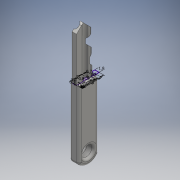
# Autodesk Inventor part: kms01
Saved by Autodesk Inventor 2016 (Build 200138000, 138)
## iProperties
Created: 2016-08-11
Part Number: kms01
Material: Generic
Document SubType Name: Modeling
Designer: Chris
Density: 1 g/cm^3
Appearance: Default
Author: Chris
Autodesk Inventor part; units mm, degrees
ref_plane "YZ Plane" through (0, 0, 0) normal (1, 0, 0) x (0, 1, 0)
ref_plane "XZ Plane" through (0, 0, 0) normal (0, 1, 0) x (-1, 0, 0)
ref_plane "XY Plane" through (0, 0, 0) normal (0, 0, 1) x (1, 0, 0)
sketch "Sketch1" plane through (0, 0, 0) normal (0, 0, 1) x (1, 0, 0)
  line L0 (-0.9, 0) -> (0.9, 0)
  line L1 (0.9, 0) -> (0.9, 9.3)
  line L2 (0.9, 9.3) -> (-0.9, 9.3)
  line L3 (-0.9, 9.3) -> (-0.9, 0)
  arc A0 (-0.9, 0.7) -> (-0.9, 2.8) centre (-0.8511, 1.75) ccw
  arc A1 (0.9, 5) -> (0.9, 3) centre (0.9, 4) ccw
  arc A2 (-0.9, 5) -> (-0.3932, 7) centre (-0.876, 6.0581) ccw
  line L4 (0.9, 7) -> (0.4, 7)
  line L5 (0.4, 7) -> (0.9, 6)
  line L6 (0.4, 7) -> (0.4, 8)
  line L7 (0.4, 8) -> (0.9, 8)
  line L8 (-0.9, 8) -> (-0.3, 8)
  line L9 (-0.3, 8) -> (-0.3, 6.9461)
  point P0 (0, 0)
  point P1 (0, 0)
  point P2 (0.2, 1.75)
  point P3 (-0.1, 4)
  point P4 (0.15, 5.7981)
  dimension "d0" = 1.8
  dimension "d1" = 9.3
  dimension "d18" = 2.8
  dimension "d19" = 0.7
  dimension "d20" = 0.7
  dimension "d21" = 3
  dimension "d22" = 5
  dimension "d23" = 0.8
  dimension "d24" = 5
  dimension "d25" = 7
  dimension "d26" = 0.75
  dimension "d27" = 7
  dimension "d28" = 6
  dimension "d29" = 0.5
  dimension "d34" = 0.7
  dimension "d35" = 8
  constraints: 20 end point, 11 point on line, 10 point on circle, 3 centre point, 3 perpendicular, 2 horizontal, 2 parallel, 1 coincident, 1 midpoint, 1 vertical
  measures "d0" distance of L2.end L1.end
  measures "d1" distance of L0.end L1.end
  measures "d18" distance from line of L0 A0.end
  measures "d19" distance of L0.start A0.start
  measures "d20" distance from line of L1 point (0.2, 1.75)
  measures "d21" distance from line of L0 A1.end
  measures "d22" distance from line of L0 A1.start
  measures "d23" distance from line of L3 point (-0.1, 4)
  measures "d24" vertical distance of point (0, 0) A2.start
  measures "d25" vertical distance of point (0, 0) A2.end
  measures "d26" distance from line of L1 point (0.15, 5.798)
  measures "d27" vertical distance of point (0, 0) L4.start
  measures "d28" vertical distance of point (0, 0) L5.end
  measures "d29" distance of L4.start L4.end
  measures "d34" distance between parallel lines of L6 L9
  measures "d35" distance from line of point (0, 0) L7
sketch "Sketch2" plane through (0, 0, 0) normal (1, 0, 0) x (0, 1, 0)
  line L0 (6.8, 0) -> (6.8, 3.6)
  line L1 (6.8, 3.6) -> (5.5, 4.9)
  line L2 (6, 17.75) -> (2.75, 21)
  line L3 (2.75, 21) -> (0, 18.25)
  line L4 (0, 18.25) -> (0, 0)
  line L5 (0, 0) -> (6.8, 0)
  line L6 (6, 16.5) -> (0, 16.5) construction
  line L7 (4.55, 13) -> (0, 13) construction
  line L8 (6.35, 9.5) -> (0, 9.5) construction
  line L9 (5.5, 6) -> (0, 6) construction
  arc A0 (3.4571, 20.2929) -> (2.0429, 20.2929) centre (2.75, 19.5858) ccw
  line L10 (5.5, 7.325) -> (5.5, 4.9)
  line L11 (6.35, 10.35) -> (6.35, 8.175)
  line L12 (4.55, 14.025) -> (4.55, 12.15)
  line L13 (6, 17.75) -> (6, 15.475)
  line L14 (6, 15.475) -> (4.55, 14.025)
  line L15 (4.55, 12.15) -> (6.35, 10.35)
  line L16 (6.35, 8.175) -> (5.5, 7.325)
  line L17 (1.375, 6) -> (1.375, 9.5) construction
  line L18 (1.375, 9.5) -> (1.375, 13) construction
  line L19 (1.375, 13) -> (1.375, 9.5) construction
  line L20 (1.375, 13) -> (1.375, 16.5) construction
  line L21 (1.375, 6) -> (1.375, 2.5) construction
  point P0 (1.375, 11.25)
  point P1 (1.375, 7.75)
  point P2 (5.45, 11.25)
  point P3 (5.925, 7.75)
  point P4 (5.275, 14.75)
  point P5 (1.375, 14.75)
  point P6 (6.15, 4.25)
  point P7 (1.375, 4.25)
  dimension "d3" = 135
  dimension "d6" = 6.8
  dimension "d7" = 5.5
  dimension "d8" = 6.35
  dimension "d9" = 4.55
  dimension "d10" = 6
  dimension "d11" = 6
  dimension "d12" = 9.5
  dimension "d13" = 13
  dimension "d14" = 16.5
  dimension "d15" = 21
  dimension "d16" = 2.75
  dimension "d17" = 1
  dimension "d39" = 135
  constraints: 48 end point, 16 point on line, 9 midpoint, 6 perpendicular, 6 vertical, 4 horizontal alignment, 4 parallel, 2 point on circle, 2 tangent, 1 centre point, 1 collinear, 1 horizontal
  measures "d3" angle of L1 L0
  measures "d6" distance between parallel lines of L4 L0
  measures "d7" distance of L9.end L9.start
  measures "d8" distance of L8.end L8.start
  measures "d9" distance of L7.end L7.start
  measures "d10" distance of L6.end L6.start
  measures "d11" distance from line of L9 L4.end
  measures "d12" distance from line of L4.end L8
  measures "d13" distance from line of L4.end L7
  measures "d14" distance from line of L4.end L6
  measures "d15" vertical distance of L4.end L2.end
  measures "d16" distance from line of L2.end L4
  measures "d17" radius of A0
  measures "d39" angle of L10 L16
extrude "Extrusion1" add sketch "Sketch1" along normal up to surface (21 mm away) contours L3 A0 A2 L9 L8 L2 L1 L7 L6 L5 A1 L0
fillet "Fillet1" radius 1 7 edges at (0.9, 5, 10.5) (0.9, 6, 10.5) (-0.9, 2.8, 10.5) (0.9, 3, 10.5) (-0.9, 5, 10.5) (-0.3, 6.9461, 10.5) (0.4, 7, 10.5)
extrude "Extrusion2" cut sketch "Sketch2" along normal through all both and the other way through all contours L5 L4 L3 A0 L2 L13 L14 L12 L15 L11 L16 L10 L1 L0 keep common part
sketch "Sketch3" plane through (0, 0, 0) normal (0, 0, 1) x (1, 0, 0)
  line L0 (0.9, 0) -> (0.9, 5.7639) projected
  line L1 (-2, 8) -> (2, 8)
  line L2 (2, 8) -> (2, 0)
  line L3 (2, 0) -> (-2, 0)
  line L4 (-2, 0) -> (-2, 8)
  line L5 (-0.9, 0) -> (0.9, 0) projected
  line L6 (0.4, 8) -> (0.9, 8) projected
  point P0 (0, 0)
  point P1 (0.9, 3)
  point P2 (0, 0)
  dimension "d47" = 4
  constraints: 8 end point, 2 midpoint, 2 parallel, 1 collinear, 1 horizontal, 1 perpendicular
  measures "d47" distance of L1.start L1.end
extrude "Extrusion3" add sketch "Sketch3" against normal blind 30
sketch "Sketch4" plane through (-2, 0, 0) normal (-1, 0, 0) x (0, 0, 1)
  circle A0 centre (-25.25, 4) radius 2.25
  line L0 (-23, 8) -> (0, 8) construction
  line L1 (0, 8) -> (0, 0) construction
  line L2 (0, 0) -> (-23, 0) construction
  line L3 (-23, 0) -> (-23, 8) construction
  line L4 (-30, 0) -> (-30, 8) projected
  line L5 (0, 0) -> (-30, 0) projected
  line L6 (0, 8) -> (-30, 8) projected
  arc A1 (-27.8117, 8) -> (-27.8117, 0) centre (-25.25, 4) ccw
  spline S0 degree 2 poles (-17.6667, 1.662) (-17.6667, 1.6197) (-17.7089, 1.554) (-17.8263, 1.5117) (-18.0376, 1.4883) (-18.1925, 1.4883) knots 0 0 0 1 2 3 4 4 4
  spline S1 degree 2 poles (-18.1925, 1.4883) (-18.4413, 1.4883) (-18.662, 1.5258) (-18.7559, 1.6056) (-18.784, 1.6573) knots 0 0 0 1 2 3 3 3
  line L7 (-18.784, 1.6573) -> (-20.2911, 4.0188)
  line L8 (-20.2911, 4.0188) -> (-20.2911, 1.6573)
  spline S2 degree 2 poles (-20.2911, 1.6573) (-20.2911, 1.615) (-20.338, 1.554) (-20.4507, 1.5117) (-20.6432, 1.4883) (-20.7934, 1.4883) knots 0 0 0 1 2 3 4 4 4
  spline S3 degree 2 poles (-20.7934, 1.4883) (-20.939, 1.4883) (-21.1362, 1.5117) (-21.2488, 1.554) (-21.3005, 1.615) (-21.3005, 1.6573) knots 0 0 0 1 2 3 4 4 4
  line L9 (-21.3005, 1.6573) -> (-21.3005, 6.3474)
  spline S4 degree 2 poles (-21.3005, 6.3474) (-21.3005, 6.3897) (-21.2488, 6.4507) (-21.1362, 6.4883) (-20.939, 6.5117) (-20.7934, 6.5117) knots 0 0 0 1 2 3 4 4 4
  spline S5 degree 2 poles (-20.7934, 6.5117) (-20.6432, 6.5117) (-20.4507, 6.4883) (-20.338, 6.4507) (-20.2911, 6.3897) (-20.2911, 6.3474) knots 0 0 0 1 2 3 4 4 4
  line L10 (-20.2911, 6.3474) -> (-20.2911, 4.2254)
  line L11 (-20.2911, 4.2254) -> (-18.831, 6.3427)
  spline S6 degree 2 poles (-18.831, 6.3427) (-18.8028, 6.3944) (-18.7277, 6.4601) (-18.6056, 6.4977) (-18.4131, 6.5117) (-18.2629, 6.5117) knots 0 0 0 1 2 3 4 4 4
  spline S7 degree 2 poles (-18.2629, 6.5117) (-18.108, 6.5117) (-17.9061, 6.4883) (-17.7887, 6.446) (-17.7418, 6.385) (-17.7418, 6.3474) knots 0 0 0 1 2 3 4 4 4
  spline S8 degree 2 poles (-17.7418, 6.3474) (-17.7418, 6.2817) (-17.8122, 6.1408) (-17.9061, 5.9906) knots 0 0 0 1 2 2 2
  line L12 (-17.9061, 5.9906) -> (-19.277, 4.2019)
  line L13 (-19.277, 4.2019) -> (-17.784, 1.9531)
  spline S9 degree 2 poles (-17.784, 1.9531) (-17.6995, 1.7981) (-17.6667, 1.6901) (-17.6667, 1.662) knots 0 0 0 1 2 2 2
  spline S10 degree 2 poles (-11.1878, 1.6479) (-11.1878, 1.6103) (-11.23, 1.5493) (-11.3427, 1.5117) (-11.5258, 1.4883) (-11.6667, 1.4883) knots 0 0 0 1 2 3 4 4 4
  spline S11 degree 2 poles (-11.6667, 1.4883) (-11.8075, 1.4883) (-11.9906, 1.5117) (-12.0986, 1.5493) (-12.1455, 1.6103) (-12.1455, 1.6479) knots 0 0 0 1 2 3 4 4 4
  line L14 (-12.1455, 1.6479) -> (-12.1455, 5.6995)
  line L15 (-12.1455, 5.6995) -> (-12.1549, 5.6995)
  line L16 (-12.1549, 5.6995) -> (-13.5962, 1.6526)
  spline S12 degree 2 poles (-13.5962, 1.6526) (-13.6103, 1.6056) (-13.6808, 1.5399) (-13.7981, 1.4977) (-13.9859, 1.4883) (-14.1174, 1.4883) knots 0 0 0 1 2 3 4 4 4
  spline S13 degree 2 poles (-14.1174, 1.4883) (-14.2441, 1.4883) (-14.4319, 1.507) (-14.5493, 1.5493) (-14.6197, 1.6103) (-14.6291, 1.6526) knots 0 0 0 1 2 3 4 4 4
  line L17 (-14.6291, 1.6526) -> (-16.0235, 5.6995)
  line L18 (-16.0235, 5.6995) -> (-16.0329, 5.6995)
  line L19 (-16.0329, 5.6995) -> (-16.0329, 1.6479)
  spline S14 degree 2 poles (-16.0329, 1.6479) (-16.0329, 1.6103) (-16.0751, 1.5493) (-16.1925, 1.5117) (-16.3709, 1.4883) (-16.5117, 1.4883) knots 0 0 0 1 2 3 4 4 4
  spline S15 degree 2 poles (-16.5117, 1.4883) (-16.6526, 1.4883) (-16.8357, 1.5117) (-16.9484, 1.5493) (-16.9906, 1.6103) (-16.9906, 1.6479) knots 0 0 0 1 2 3 4 4 4
  line L20 (-16.9906, 1.6479) -> (-16.9906, 6.0845)
  spline S16 degree 2 poles (-16.9906, 6.0845) (-16.9906, 6.2817) (-16.784, 6.4883) (-16.6103, 6.4883) knots 0 0 0 1 2 2 2
  line L21 (-16.6103, 6.4883) -> (-15.9484, 6.4883)
  spline S17 degree 2 poles (-15.9484, 6.4883) (-15.77, 6.4883) (-15.5164, 6.4319) (-15.3333, 6.2958) (-15.2113, 6.0751) (-15.1643, 5.9155) knots 0 0 0 1 2 3 4 4 4
  line L22 (-15.1643, 5.9155) -> (-14.0845, 2.9484)
  line L23 (-14.0845, 2.9484) -> (-14.0704, 2.9484)
  line L24 (-14.0704, 2.9484) -> (-12.9531, 5.9061)
  spline S18 degree 2 poles (-12.9531, 5.9061) (-12.9014, 6.0704) (-12.784, 6.2911) (-12.6244, 6.4319) (-12.4131, 6.4883) (-12.2676, 6.4883) knots 0 0 0 1 2 3 4 4 4
  line L25 (-12.2676, 6.4883) -> (-11.5869, 6.4883)
  spline S19 degree 2 poles (-11.5869, 6.4883) (-11.4836, 6.4883) (-11.3333, 6.4366) (-11.2394, 6.3286) (-11.1878, 6.1784) (-11.1878, 6.0845) knots 0 0 0 1 2 3 4 4 4
  line L26 (-11.1878, 6.0845) -> (-11.1878, 1.6479)
  spline S20 degree 2 poles (-7.1549, 3.0047) (-7.1549, 2.6103) (-7.446, 2.0188) (-7.9484, 1.6244) (-8.615, 1.4225) (-8.9953, 1.4225) knots 0 0 0 1 2 3 4 4 4
  spline S21 degree 2 poles (-8.9953, 1.4225) (-9.2535, 1.4225) (-9.6948, 1.507) (-10.0329, 1.6291) (-10.2629, 1.7606) (-10.3615, 1.8592) (-10.4038, 2.0469) (-10.4038, 2.2254) knots 0 0 0 1 2 3 4 5 6 6 6
  spline S22 degree 2 poles (-10.4038, 2.2254) (-10.4038, 2.3427) (-10.3897, 2.507) (-10.3521, 2.6056) (-10.2958, 2.6479) (-10.2582, 2.6479) knots 0 0 0 1 2 3 4 4 4
  spline S23 degree 2 poles (-10.2582, 2.6479) (-10.2019, 2.6479) (-10.0094, 2.5211) (-9.6995, 2.3662) (-9.2723, 2.2394) (-8.9953, 2.2394) knots 0 0 0 1 2 3 4 4 4
  spline S24 degree 2 poles (-8.9953, 2.2394) (-8.8075, 2.2394) (-8.5164, 2.3286) (-8.3146, 2.4883) (-8.2066, 2.7277) (-8.2066, 2.8732) knots 0 0 0 1 2 3 4 4 4
  spline S25 degree 2 poles (-8.2066, 2.8732) (-8.2066, 3.0423) (-8.3897, 3.2864) (-8.6854, 3.4742) (-9.061, 3.6385) (-9.4648, 3.8216) (-9.8404, 4.0563) (-10.1362, 4.385) (-10.3192, 4.831) (-10.3192, 5.1408) knots 0 0 0 1 2 3 4 5 6 7 8 8 8
  spline S26 degree 2 poles (-10.3192, 5.1408) (-10.3192, 5.5023) (-10.0516, 6.0423) (-9.6056, 6.3991) (-8.9906, 6.5775) (-8.6479, 6.5775) knots 0 0 0 1 2 3 4 4 4
  spline S27 degree 2 poles (-8.6479, 6.5775) (-8.4742, 6.5775) (-8.1174, 6.5258) (-7.8122, 6.4319) (-7.5728, 6.3146) (-7.493, 6.2394) (-7.4695, 6.1878) (-7.4507, 6.0986) (-7.4413, 5.9624) (-7.4413, 5.8638) knots 0 0 0 1 2 3 4 5 6 7 8 8 8
  spline S28 degree 2 poles (-7.4413, 5.8638) (-7.4413, 5.7512) (-7.4507, 5.5962) (-7.4789, 5.4977) (-7.5305, 5.4507) (-7.5728, 5.4507) knots 0 0 0 1 2 3 4 4 4
  spline S29 degree 2 poles (-7.5728, 5.4507) (-7.615, 5.4507) (-7.7981, 5.5587) (-8.0704, 5.6854) (-8.4225, 5.7887) (-8.6338, 5.7887) knots 0 0 0 1 2 3 4 4 4
  spline S30 degree 2 poles (-8.6338, 5.7887) (-8.7981, 5.7887) (-9.0469, 5.7089) (-9.2113, 5.5634) (-9.2911, 5.3662) (-9.2911, 5.2535) knots 0 0 0 1 2 3 4 4 4
  spline S31 degree 2 poles (-9.2911, 5.2535) (-9.2911, 5.0892) (-9.1127, 4.8451) (-8.8075, 4.6573) (-8.4225, 4.493) (-8.0235, 4.3099) (-7.6385, 4.0751) (-7.338, 3.7465) (-7.1549, 3.3052) (-7.1549, 3.0047) knots 0 0 0 1 2 3 4 5 6 7 8 8 8
  spline S32 degree 2 poles (-1.5117, 1.8967) (-1.5117, 1.7887) (-1.5352, 1.6385) (-1.5775, 1.5493) (-1.6291, 1.5117) (-1.6667, 1.5117) knots 0 0 0 1 2 3 4 4 4
  line L27 (-1.6667, 1.5117) -> (-4.4131, 1.5117)
  spline S33 degree 2 poles (-4.4131, 1.5117) (-4.446, 1.5117) (-4.4977, 1.5493) (-4.5399, 1.6385) (-4.5634, 1.7887) (-4.5634, 1.8967) knots 0 0 0 1 2 3 4 4 4
  spline S34 degree 2 poles (-4.5634, 1.8967) (-4.5634, 2.0047) (-4.5446, 2.1549) (-4.5023, 2.2488) (-4.446, 2.2911) (-4.4131, 2.2911) knots 0 0 0 1 2 3 4 4 4
  line L28 (-4.4131, 2.2911) -> (-3.4883, 2.2911)
  line L29 (-3.4883, 2.2911) -> (-3.4883, 5.5352)
  line L30 (-3.4883, 5.5352) -> (-4.2911, 5.0939)
  spline S35 degree 2 poles (-4.2911, 5.0939) (-4.3756, 5.0516) (-4.4883, 5.0329) (-4.554, 5.0986) (-4.5775, 5.2582) (-4.5775, 5.4038) knots 0 0 0 1 2 3 4 4 4
  spline S36 degree 2 poles (-4.5775, 5.4038) (-4.5775, 5.4977) (-4.5681, 5.615) (-4.5399, 5.6995) (-4.4836, 5.7559) (-4.4366, 5.784) knots 0 0 0 1 2 3 4 4 4
  line L31 (-4.4366, 5.784) -> (-3.3709, 6.4742)
  spline S37 degree 2 poles (-3.3709, 6.4742) (-3.3474, 6.493) (-3.2911, 6.5117) (-3.1972, 6.5211) (-3.0469, 6.5258) (-2.9296, 6.5258) knots 0 0 0 1 2 3 4 4 4
  spline S38 degree 2 poles (-2.9296, 6.5258) (-2.784, 6.5258) (-2.6009, 6.5164) (-2.5117, 6.4883) (-2.4789, 6.4413) (-2.4789, 6.4085) knots 0 0 0 1 2 3 4 4 4
  line L32 (-2.4789, 6.4085) -> (-2.4789, 2.2911)
  line L33 (-2.4789, 2.2911) -> (-1.6667, 2.2911)
  spline S39 degree 2 poles (-1.6667, 2.2911) (-1.6291, 2.2911) (-1.5728, 2.2488) (-1.5305, 2.1549) (-1.5117, 2.0047) (-1.5117, 1.8967) knots 0 0 0 1 2 3 4 4 4
  point P0 (0, -4.2458)
  point P1 (-30, 4)
  point P2 (-30, 4)
  dimension "d40" = 4.5
  dimension "d48" = 2.5
  constraints: 3 point on circle, 3 point on line, 2 centre point, 2 coincident, 2 midpoint, 2 tangent, 1 horizontal, 1 horizontal alignment, 2 other
  measures "d40" diameter of A0
  measures "d48" radial gap between concentric circles of A1 A0
emboss "Emboss1" sketch "Sketch4" operation cut depth 0.5 direction (1, 0, 0) contours S0 S1 L7 L8 S2 S3 L9 S4 S5 L10 L11 S6 S7 S8 L12 L13 S9 | S10 S11 L14 L15 L16 S12 S13 L17 L18 L19 S14 S15 L20 S16 L21 S17 L22 L23 L24 S18 L25 S19 L26 | S20 S21 S22 S23 S24 S25 S26 S27 S28 S29 S30 S31 | S32 L27 S33 S34 L28 L29 L30 S35 S36 L31 S37 S38 L32 L33 S39
extrude "Extrusion4" cut sketch "Sketch4" against normal through all contours A0 | L4 L6 A1 | L4 A1 L5
fillet "Fillet2" radius 1 13 edges at (2, 4, -27.5) (-2, 4, -27.5) (-2, 4, -30) (2, 4, -30) (2, 8, -13.9059) (-2, 8, -13.9059) (0, 8, -27.8117) (0, 0, -27.8117) (-2, 0, -13.9059) (2, 0, -13.9059) (-2, 4, 0) (0, 8, 0) (2, 4, 0)
equation "\"d39\" = d3"
body "Solid1"
